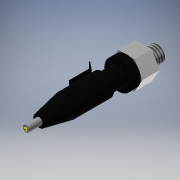
# Autodesk Inventor part: 30PSIPressureSensor
Saved by Autodesk Inventor 2016 (Build 200138000, 138)
## iProperties
Created: 2015-11-21
Part Number: 30PSIPressureSensor
Material: Generic
Document SubType Name: Modeling
Designer: al11g09
Density: 1 g/cm^3
Appearance: Default
Author: al11g09
Autodesk Inventor part; units mm, degrees
ref_plane "YZ Plane" through (0, 0, 0) normal (1, 0, 0) x (0, 1, 0)
ref_plane "XZ Plane" through (0, 0, 0) normal (0, 1, 0) x (-1, 0, 0)
ref_plane "XY Plane" through (0, 0, 0) normal (0, 0, 1) x (1, 0, 0)
sketch "Sketch1" plane through (0, 0, 0) normal (0, 0, 1) x (1, 0, 0)
  line L0 (0, 13.8093) -> (0, -15.119)
  line L1 (0, 0) -> (10.75, 0)
  line L2 (10.75, 0) -> (10.75, -6)
  line L3 (10.75, -6) -> (6.65, -6)
  line L4 (6.65, -6) -> (6.65, -18)
  line L5 (6.65, -18) -> (8.5, -18)
  line L6 (8.5, -18) -> (8.5, -46)
  line L7 (8.5, -46) -> (4.5, -66)
  line L8 (4.5, -66) -> (0, -66)
  line L9 (0, -66) -> (0, 0)
  dimension "d0" = 10.75
  dimension "d1" = 6
  dimension "d2" = 4.1
  dimension "d3" = 12
  dimension "d4" = 28
  dimension "d5" = 1.85
  dimension "d6" = 20
  dimension "d7" = 4.5
  constraints: 20 end point, 3 horizontal, 3 vertical, 2 perpendicular, 1 collinear, 1 point on line
  measures "d0" distance of L1.start L1.end
  measures "d1" distance of L1.end L2.end
  measures "d2" distance of L2.end L3.end
  measures "d3" distance of L3.end L4.end
  measures "d4" distance of L5.end L6.end
  measures "d5" distance of L4.end L5.end
  measures "d6" vertical distance of L7.end L6.end
  measures "d7" distance of L7.end L8.end
revolve "body" add sketch "Sketch1" angle 360 about axis through (0, 13.8093, 0) along (0, -1, 0)
sketch "Sketch2" plane through (0, 0, 0) normal (0, 1, 0) x (-1, 0, 0)
  circle A0 centre (0, 0) radius 6.65 construction
  circle A1 centre (0, 0) radius 12.2 construction
  line L0 (6.1, -10.5655) -> (-6.1, -10.5655)
  line L1 (-6.1, -10.5655) -> (-12.2, 0)
  line L2 (12.2, 0) -> (-12.2, 0) construction
  line L3 (-12.2, 0) -> (-6.1, 10.5655)
  line L4 (6.1, 10.5655) -> (-6.1, 10.5655)
  line L5 (6.1, 10.5655) -> (12.2, 0)
  line L6 (12.2, 0) -> (6.1, -10.5655)
  point P0 (0, 0)
  dimension "d9" = 24.4
  constraints: 14 end point, 3 horizontal, 2 equal length, 1 coincident, 1 midpoint, 1 point on line, 9 other
extrude "hexBit" add sketch "Sketch2" along normal blind 13
sketch "Sketch3" plane through (0, 0, 0) normal (0, 0, 1) x (1, 0, 0)
  line L0 (-6.1, 13) -> (6.1, 13) construction
  line L1 (-6.1, 13) -> (-6.1, 23)
  line L2 (-6.1, 23) -> (-1.5, 23)
  line L3 (-1.5, 23) -> (-1.5, 15)
  line L4 (6.1, 13) -> (-6.1, 13) projected
  line L5 (0, 13) -> (0, 41.9398)
  line L6 (-6.1, 13) -> (0, 13)
  line L7 (0, 13) -> (0, 15)
  line L8 (0, 15) -> (-1.5, 15)
  point P0 (0, 0)
  dimension "d12" = 10
  dimension "d14" = 8
  dimension "d17" = 1.5
  constraints: 14 end point, 3 vertical, 2 perpendicular, 1 collinear, 1 midpoint, 1 point on line
  measures "d12" distance of L0.start L1.end
  measures "d14" distance of L2.end L3.end
  measures "d17" distance of L7.end L3.end
revolve "sensorENtrance" add sketch "Sketch3" angle 360 about axis through (0, 13, 0) along (0, 1, 0)
thread "Thread1" size "M14x2" class "6g" standard "ANSI Metric M Profile" full length
sketch "Sketch5" plane through (0, 0, 0) normal (0, 0, 1) x (1, 0, 0)
  line L0 (-8.5, -46) -> (8.5, -46) construction
  line L1 (-8.5, -18) -> (8.5, -18) construction
  line L2 (-8.5, -34) -> (-9.5, -34)
  line L3 (-9.5, -34) -> (-9.5, -18)
  line L4 (-8.5, -18) -> (-8.5, -46) projected
  line L5 (-9.5, -18) -> (-14.5, -14)
  line L6 (-8.5, -18) -> (-8.5, -34)
  line L7 (-8.5, -18) -> (8.5, -18) projected
  line L8 (-13.5, -14) -> (-8.5, -18)
  line L9 (-14.5, -14) -> (-13.5, -14)
  point P0 (0, 0)
  dimension "d21" = 1
  dimension "d22" = 16
  dimension "d24" = 4
  dimension "d25" = 5
  constraints: 12 end point, 3 point on line, 2 horizontal, 2 parallel, 1 vertical
  measures "d21" distance of L2.start L2.end
  measures "d22" distance of L2.end L3.end
  measures "d24" vertical distance of L5.end L3.end
  measures "d25" horizontal distance of L3.end L5.end
extrude "stickingOutBit" add sketch "Sketch5" along normal mid plane 12
sketch "Sketch6" plane through (0, -66, 0) normal (0, -1, 0) x (1, 0, 0)
  circle A0 centre (0, 0) radius 2.5
  dimension "d28" = 5
  constraints: 1 centre point, 1 coincident
  measures "d28" diameter of A0
extrude "lead" add sketch "Sketch6" along normal blind 10
sketch "pinsPlacement" plane through (0, -76, 0) normal (0, -1, 0) x (1, 0, 0)
  line L0 (-1.2888, 0) -> (1.0188, 0) construction
  line L1 (0.5, 0.75) -> (0.5, -0.75) construction
  point P0 (0, 0)
  point P1 (-0.75, 0)
  point P2 (0.5, 0)
  dimension "d31" = 0.75
  dimension "d32" = 0.5
  dimension "d33" = 1.5
  constraints: 4 end point, 3 point on line, 1 horizontal, 1 midpoint, 1 vertical
  measures "d31" distance of point (0, 0) point (-0.75, 0)
  measures "d32" distance from line of point (0, 0) L1
  measures "d33" diameter of L1.start L0
body "Solid1"
